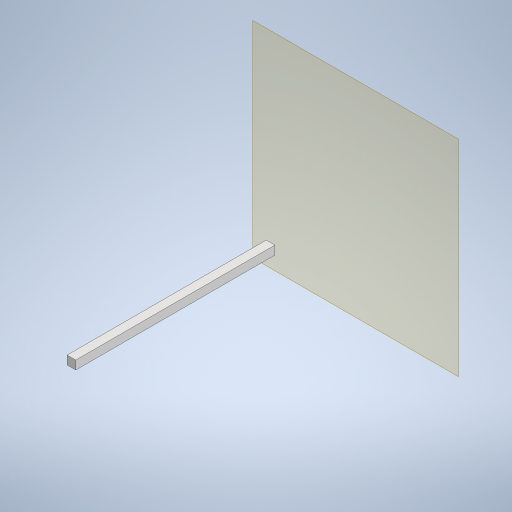
# Autodesk Inventor part: BarraVertical
Saved by Autodesk Inventor 2024 (Build 280153000, 153)
## iProperties
Created: 2023-06-26
Part Number: BarraVertical
Material: Genérico
Document SubType Name: Modeling
Designer: Personal
Density: 2.87828 g/cm^3
Appearance: Valor por defecto
Mass: 48.4 g
Surface Area: 76.356 cm^2
Volume: 16.8156 cm^3
Author: Personal
Autodesk Inventor part; units mm, degrees
ref_plane "YZ Plane" through (0, 0, 0) normal (1, 0, 0) x (0, 1, 0)
ref_plane "XZ Plane" through (0, 0, 0) normal (0, 1, 0) x (-1, 0, 0)
ref_plane "XY Plane" through (0, 0, 0) normal (0, 0, 1) x (1, 0, 0)
ref_plane "Plano de trabajo1" through (0, 0, 0) normal (0, 0, 1) x (1, 0, 0)
sketch "Boceto1" plane through (0, 0, 0) normal (0, 0, 1) x (1, 0, 0)
  line L0 (-93.1, -97.5) -> (-93.1, 97.5) construction
  line L1 (93.1, -93.1) -> (-93.1, -93.1) construction
  line L2 (-93.1, -93.1) -> (-84.1, -93.1) construction
  line L3 (-84.1, -93.1) -> (-84.1, -84.1)
  line L4 (-84.1, -84.1) -> (-93.1, -84.1)
  line L5 (-93.1, -84.1) -> (-93.1, -93.1) construction
  line L6 (-93.1, -93.1) -> (-84.1, -93.1)
  line L7 (-93.1, -93.1) -> (-93.1, -84.1)
  point P0 (0, 0)
  dimension "d2" = 9
  dimension "d3" = 9
  constraints: 12 end point, 2 collinear, 2 parallel, 1 horizontal, 1 perpendicular
  measures "d2" distance of L2.end L3.end
  measures "d3" distance of L3.end L4.end
extrude "Extrusión1" add sketch "Boceto1" along normal blind 207.6
